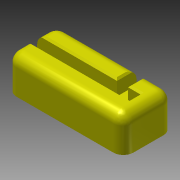
# Autodesk Inventor part: Apoyo frontal
Saved by Autodesk Inventor 2014 (Build 180170000, 170)
## iProperties
Created: 2016-10-07
Part Number: Apoyo frontal
Material: Generic
Document SubType Name: Modeling
Designer: Rubén
Density: 1 g/cm^3
Appearance: Smooth - Yellow
Author: Rubén
Autodesk Inventor part; units mm, degrees
ref_plane "YZ Plane" through (0, 0, 0) normal (1, 0, 0) x (0, 1, 0)
ref_plane "XZ Plane" through (0, 0, 0) normal (0, 1, 0) x (-1, 0, 0)
ref_plane "XY Plane" through (0, 0, 0) normal (0, 0, 1) x (1, 0, 0)
sketch "Sketch1" plane through (0, 0, 0) normal (0, 1, 0) x (-1, 0, 0)
  line L0 (0, 0) -> (35, 0)
  line L1 (35, 0) -> (35, 15)
  line L2 (35, 15) -> (0, 15)
  line L3 (0, 15) -> (0, 0)
  dimension "d0" = 35
  dimension "d1" = 15
  constraints: 8 end point, 2 parallel, 1 horizontal, 1 perpendicular
  measures "d0" distance of L2.end L1.end
  measures "d1" distance of L1.end L0.end
extrude "Extrusion1" add sketch "Sketch1" along normal blind 4
sketch "Sketch2" plane through (0, 4, 0) normal (0, 1, 0) x (1, 0, 0)
  line L0 (0, 0) -> (-35, 0) projected
  line L1 (-35, 0) -> (-35, -15) projected
  line L2 (-35, -15) -> (0, -15) projected
  line L3 (0, -15) -> (0, 0) projected
  line L4 (-35, -5.85) -> (-31, -5.85)
  line L5 (-35, -9.15) -> (0, -9.15)
  line L6 (-17.5, -15) -> (-17.5, -9.15) construction
  line L7 (-17.5, -5.85) -> (-17.5, 0) construction
  line L8 (-31, -5.85) -> (-31, -9.15)
  line L9 (-4, -5.85) -> (-4, -9.15)
  line L10 (-4, -5.85) -> (0, -5.85)
  line L11 (-31, -5.85) -> (-4, -5.85)
  dimension "d4" = 3.3
  dimension "d7" = 27
  constraints: 16 end point, 6 perpendicular, 6 point on line, 4 midpoint, 2 collinear, 1 parallel
  measures "d4" distance between parallel lines of L5 L4
  measures "d7" distance between parallel lines of L9 L8
extrude "Extrusion2" add sketch "Sketch2" along normal blind 2 contours L3 L10 L11 L4 L1 L0 | L3 L5 L9 L10 | L4 L8 L5 L1 | L3 L2 L1 L5
sketch "Sketch3" plane through (0, 6, 0) normal (0, 1, 0) x (1, 0, 0)
  line L0 (0, -15) -> (0, 0) projected
  line L1 (0, 0) -> (-35, 0) projected
  line L2 (-35, 0) -> (-35, -15) projected
  line L3 (-35, -15) -> (0, -15) projected
  line L4 (-4, -9.15) -> (-31, -9.15) projected
  line L5 (-31, -9.15) -> (-31, -5.85) projected
  line L6 (-31, -5.85) -> (-4, -5.85) projected
  line L7 (-4, -5.85) -> (-4, -9.15) projected
  line L8 (-31, -5.85) -> (-35, -5.85)
  line L9 (-31, -9.15) -> (-35, -9.15)
  line L10 (-7.75, -5.85) -> (-7.75, 0)
  line L11 (-11.05, -5.85) -> (-11.05, 0)
  line L12 (-11.05, -2.925) -> (-7.75, -2.925) construction
  dimension "d16" = 3.75
  constraints: 10 end point, 6 point on line, 4 perpendicular, 2 midpoint, 1 parallel
  measures "d16" distance between parallel lines of L10 L7
extrude "Extrusion3" add sketch "Sketch3" along normal blind 4.5 contours L3 L2 L9 L4 L7 L6 L10 L1 L0 | L11 L6 L8 L2 L1
chamfer "Chamfer3" distance 2 angle 45 1 edges at (-31, 4, 7.5)
fillet "Fillet3" radius 3 1 edges at (-4, 4, 7.5)
chamfer "Chamfer2" distance 0.5 angle 45 6 edges at (-19.5, 10.5, 9.15) (-23.025, 10.5, 5.85) (-5.875, 10.5, 5.85) (-4, 10.5, 7.5) (-7.75, 10.5, 2.925) (-11.05, 10.5, 2.925)
fillet "Fillet2" radius 3 10 edges at (0, 5.25, 15) (0, 5.25, 0) (-35, 5.25, 15) (-35, 5.25, 0) (-3.625, 10.5, 0) (0, 10.5, 7.5) (-17.5, 10.5, 15) (-23.275, 10.5, 0) (-35, 10.5, 2.675) (-35, 10.5, 12.325)
body "Solid1"
